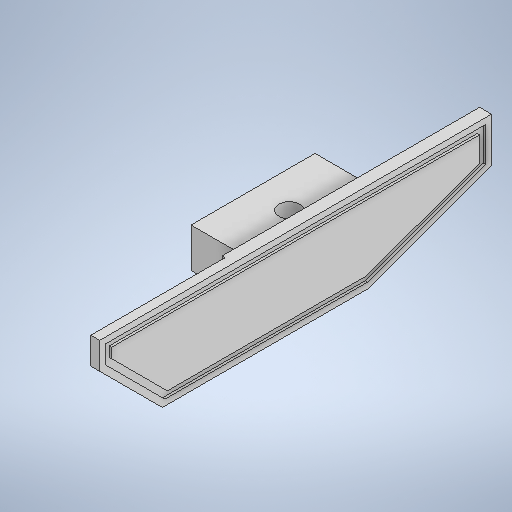
# Autodesk Inventor part: switch_cap_bl
Saved by Autodesk Inventor 2025 (Build 290162000, 162)
## iProperties
Created: 2026-08-05
Part Number: switch_cap_bl
Material: Типовые
Document SubType Name: Modeling
Designer: garin
Density: 1 g/cm^3
Appearance: По умолчанию
Author: garin
Autodesk Inventor part; units mm, degrees
ref_plane "YZ Plane" through (0, 0, 0) normal (1, 0, 0) x (0, 1, 0)
ref_plane "XZ Plane" through (0, 0, 0) normal (0, 1, 0) x (-1, 0, 0)
ref_plane "XY Plane" through (0, 0, 0) normal (0, 0, 1) x (1, 0, 0)
sketch "Эскиз1" plane through (0, 0, 0) normal (1, 0, 0) x (0, 1, 0)
  line L0 (-7.5, -32.85) -> (7.5, -32.85)
  line L1 (7.5, -32.85) -> (7.5, 32.85)
  line L2 (7.5, 32.85) -> (-7.5, 32.85)
  line L3 (-7.5, 32.85) -> (-7.5, -32.85)
  line L4 (-7.5, -32.85) -> (7.5, 32.85) construction
  line L5 (7.5, -32.85) -> (-7.5, 32.85) construction
  line L6 (0, -32.85) -> (0, -16.55) construction
  line L7 (3.3, 4.25) -> (-3.3, 4.25)
  line L8 (-3.3, 4.25) -> (-3.3, -16.55)
  line L9 (-3.3, -16.55) -> (3.3, -16.55)
  line L10 (3.3, -16.55) -> (3.3, 4.25)
  line L11 (7.5, 32.85) -> (-7.5, 32.85)
  line L12 (-7.5, 32.85) -> (-7.5, 10.35)
  line L13 (-7.5, 10.35) -> (7.5, 10.35)
  line L14 (7.5, 10.35) -> (7.5, 32.85)
  line L15 (0, -32.85) -> (-7.5, -12.2439)
  line L16 (0, -32.85) -> (21.9285, -32.85) construction
  point P0 (0, 0)
  point P1 (7.5, 10.35)
  dimension "d0" = 15
  dimension "d1" = 65.7
  dimension "d2" = 16.3
  dimension "d3" = 6.6
  dimension "d4" = 20.8
  dimension "d5" = 22.5
  dimension "d25" = 110
  constraints: 34 end point, 6 parallel, 4 horizontal, 4 midpoint, 3 perpendicular, 2 point on line, 1 equal length, 1 vertical
  measures "d0" distance of L2.end L1.end
  measures "d1" distance of L1.end L0.end
  measures "d2" distance of L6.end L6.start
  measures "d3" distance of L9.end L8.end
  measures "d4" distance of L8.end L7.end
  measures "d5" distance of L12.end L11.end
  measures "d25" angle of L16 L15
extrude "Выдавливание1" add sketch "Эскиз1" along normal blind 2 contours L15 L3 L13 L1 L0 | L3 L2 L1 L13 | L10 L9 L8 L7
extrude "Выдавливание2" add sketch "Эскиз1" against normal blind 11.3 contours L10 L9 L8 L7
extrude "Выдавливание3" cut sketch "Эскиз1" along normal blind 0.5 contours L3 L2 L1 L13
chamfer "Фаска2" distance 10.5 angle 45 1 edges at (1.25, -7.5, 32.85)
sketch "Эскиз2" plane through (2, 0, 0) normal (1, 0, 0) x (0, 0, -1)
  line L0 (-22.35, -7.5) -> (-32.85, 3) projected
  line L1 (-22.35, -7.5) -> (12.2439, -7.5) projected
  line L2 (32.85, 0) -> (32.85, 7.5) projected
  line L3 (32.85, 7.5) -> (-32.85, 7.5) projected
  line L4 (-32.85, 7.5) -> (-32.85, 3) projected
  line L5 (12.2439, -7.5) -> (32.85, 0) projected
  line L6 (31.85, 0.7002) -> (12.0676, -6.5)
  line L7 (12.0676, -6.5) -> (-21.9358, -6.5)
  line L8 (-21.9358, -6.5) -> (-31.85, 3.4142)
  line L9 (-31.85, 3.4142) -> (-31.85, 6.5)
  line L10 (-31.85, 6.5) -> (31.85, 6.5)
  line L11 (31.85, 6.5) -> (31.85, 0.7002)
  line L12 (30.85, 5.5) -> (-30.85, 5.5)
  line L13 (-30.85, 5.5) -> (-30.85, 3.8284)
  line L14 (-30.85, 3.8284) -> (-21.5216, -5.5)
  line L15 (-21.5216, -5.5) -> (11.8913, -5.5)
  line L16 (11.8913, -5.5) -> (30.85, 1.4004)
  line L17 (30.85, 1.4004) -> (30.85, 5.5)
  point P0 (0, 0)
  dimension "d26" = 1
  dimension "d32" = 1
  constraints: 24 end point, 10 other
  measures "d26" distance between parallel lines of L5 L6
  measures "d32" distance between parallel lines of L10 L12
extrude "Выдавливание5" cut sketch "Эскиз2" against normal blind 0.4 contours L6 L7 L8 L9 L10 L11
sketch "Эскиз3" plane through (-11.3, 3.3, -16.55) normal (0, 1, 0) x (1, 0, 0)
  line L0 (0, 0) -> (0, -20.8) projected
  line L1 (0, 0) -> (6.1, 0) construction
  line L2 (6.1, 0) -> (6.1, -10.4) construction
  line L3 (6.1, -10.4) -> (0, -10.4) construction
  line L4 (0, -10.4) -> (0, 0) construction
  circle A0 centre (6.1, -10.4) radius 1.75
  point P0 (11.3, -16.55)
  dimension "d27" = 6.1
  dimension "d28" = 10.4
  dimension "d29" = 3.5
  constraints: 8 end point, 2 parallel, 1 centre point, 1 coincident, 1 horizontal, 1 perpendicular
  measures "d27" distance of L2.end L3.end
  measures "d28" distance of L1.end L2.end
  measures "d29" diameter of A0
extrude "Выдавливание6" cut sketch "Эскиз3" against normal blind 5
